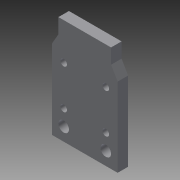
# Autodesk Inventor part: Arm_Link_Shim_i
Saved by Autodesk Inventor 2013 (Build 170138000, 138)
## iProperties
Created: 2014-05-19
Part Number: Arm_Link_Shim_i
Material: 一般
Document SubType Name: Modeling
Designer: andou
Density: 1 g/cm^3
Mass: 3.66423 g
Surface Area: 25.6367 cm^2
Volume: 3.66423 cm^3
Author: andou
Autodesk Inventor part; units mm, degrees
ref_plane "YZ Plane" through (0, 0, 0) normal (1, 0, 0) x (0, 1, 0)
ref_plane "XZ Plane" through (0, 0, 0) normal (0, 1, 0) x (-1, 0, 0)
ref_plane "XY Plane" through (0, 0, 0) normal (0, 0, 1) x (1, 0, 0)
sketch "スケッチ1" plane through (0, 0, 0) normal (0, 1, 0) x (-1, 0, 0)
  line L0 (-12.5, 20) -> (12.5, 20)
  line L1 (12.5, 20) -> (12.5, -20)
  line L2 (12.5, -20) -> (-12.5, -20)
  line L3 (-12.5, -20) -> (-12.5, 20)
  point P0 (0, 0)
  dimension "d0" = 25
  dimension "d2" = 40
  dimension "d3" = 20
  dimension "d4" = 12.5
  constraints: 8 end point, 2 parallel, 1 horizontal, 1 perpendicular
  measures "d0" distance of L0.start L0.end
  measures "d2" distance of L2.end L0.start
  measures "d3" distance from line of L0 point (0, 0)
  measures "d4" distance from line of L1 point (0, 0)
extrude "押し出し1" add sketch "スケッチ1" along normal blind 4
sketch "スケッチ2" plane through (0, 4, 0) normal (0, 1, 0) x (1, 0, 0)
  line L0 (-12.5, -20) -> (12.5, -20) projected
  line L1 (12.5, -20) -> (12.5, 20) projected
  line L2 (12.5, 20) -> (-12.5, 20) projected
  line L3 (-12.5, 20) -> (-12.5, -20) projected
  line L4 (-12.5, -10) -> (-10, -14.3301)
  line L5 (-10, -14.3301) -> (-10, -20)
  line L6 (10, -14.3301) -> (10, -20)
  line L7 (10, -14.3301) -> (12.5, -10)
  point P0 (0, 0)
  dimension "d7" = 20
  dimension "d9" = 2.5
  dimension "d10" = 30
  dimension "d11" = 150
  dimension "d12" = 30
  dimension "d13" = 150
  constraints: 8 end point, 4 point on line, 1 parallel, 1 perpendicular
  measures "d7" distance between parallel lines of L6 L5
  measures "d9" distance between parallel lines of L3 L5
  measures "d10" distance from line of L2 L4.start
  measures "d11" angle of L3 L4
  measures "d12" distance of L1.end L7.end
  measures "d13" angle of L1 L7
extrude "押し出し2" cut sketch "スケッチ2" against normal blind 4 contours L5 L4 L3 L2 L1 L7 L6 L0 keep common part
sketch "スケッチ3" plane through (0, 4, 0) normal (0, 1, 0) x (1, 0, 0)
  line L0 (12.5, 20) -> (-12.5, 20) projected
  circle A0 centre (-8, 15) radius 2
  circle A1 centre (8, 15) radius 2
  point P0 (0, 0)
  dimension "d16" = 4
  dimension "d18" = 16
  dimension "d19" = 5
  dimension "d20" = 5
  dimension "d21" = 8
  constraints: 2 centre point, 1 equal radius
  measures "d16" diameter of A0
  measures "d18" distance of A1.centre A0.centre
  measures "d19" distance from line of L0 A0.centre
  measures "d20" distance from line of L0 A1.centre
  measures "d21" horizontal distance of point (0, 0) A0.centre
hole "穴1" at (-8, 4, -15) at (8, 4, -15) direction (0, -1, 0) diameter 4 end through all
sketch "スケッチ4" plane through (0, 4, 0) normal (0, 1, 0) x (1, 0, 0)
  circle A0 centre (-8, 15) radius 2 projected
  circle A1 centre (8, 15) radius 2 projected
  circle A2 centre (-8, 9) radius 1.5
  circle A3 centre (8, 9) radius 1.5
  circle A4 centre (-8, -6) radius 1.5
  circle A5 centre (8, -6) radius 1.5
  line L0 (12.5, 20) -> (-12.5, 20) projected
  point P0 (0, 0)
  dimension "d29" = 8
  dimension "d31" = 3
  dimension "d33" = 6
  dimension "d34" = 6
  dimension "d35" = 16
  dimension "d36" = 16
  dimension "d37" = 8
  dimension "d40" = 15
  dimension "d41" = 15
  dimension "d49" = 5
  constraints: 4 centre point, 3 equal radius
  measures "d29" horizontal distance of point (0, 0) A2.centre
  measures "d31" diameter of A2
  measures "d33" distance of A0.centre A2.centre
  measures "d34" distance of A1.centre A3.centre
  measures "d35" distance of A3.centre A2.centre
  measures "d36" distance of A5.centre A4.centre
  measures "d37" horizontal distance of point (0, 0) A5.centre
  measures "d40" distance of A2.centre A4.centre
  measures "d41" distance of A3.centre A5.centre
  measures "d49" distance from line of L0 A0.centre
hole "穴2" at (-8, 4, 6) at (-8, 4, -9) at (8, 4, 6) at (8, 4, -9) direction (0, -1, 0) diameter 2.5 end through all
